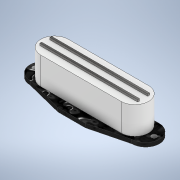
# Autodesk Inventor part: Pickup
Saved by Autodesk Inventor 2021 (Build 250183000, 183)
## iProperties
Created: 2021-02-08
Part Number: Pickup
Material: Generic
Document SubType Name: Modeling
Designer: Ryan
Density: 1 g/cm^3
Appearance: Default
Author: Ryan
Autodesk Inventor part; units mm, degrees
ref_plane "YZ Plane" through (0, 0, 0) normal (1, 0, 0) x (0, 1, 0)
ref_plane "XZ Plane" through (0, 0, 0) normal (0, 1, 0) x (-1, 0, 0)
ref_plane "XY Plane" through (0, 0, 0) normal (0, 0, 1) x (1, 0, 0)
sketch "Sketch1" plane through (0, 0, 0) normal (0, 1, 0) x (-1, 0, 0)
  line L0 (33.02, -8.89) -> (-33.02, -8.89)
  line L1 (-33.02, 8.89) -> (33.02, 8.89)
  arc A0 (33.02, -8.89) -> (33.02, 8.89) centre (33.02, 0) ccw
  arc A1 (-33.02, 8.89) -> (-33.02, -8.89) centre (-33.02, 0) ccw
  line L2 (41.91, -12.3525) -> (41.91, 10.1693) construction
  line L3 (-41.91, -12.3525) -> (-41.91, 10.1693) construction
  line L4 (8.89, 14.986) -> (-8.89, 14.986)
  line L5 (-8.89, 14.986) -> (-33.02, 8.89)
  line L6 (8.89, 14.986) -> (33.02, 8.89)
  point P0 (0, 0)
  dimension "d1" = 83.82
  dimension "d2" = 17.78
  dimension "d3" = 8.89
  dimension "d4" = 8.89
  dimension "d5" = 41.91
  dimension "d8" = 17.78
  dimension "d9" = 8.89
  dimension "d10" = 23.876
  constraints: 14 end point, 4 point on circle, 2 centre point, 2 horizontal, 2 tangent, 2 vertical, 1 equal radius, 1 parallel
  measures "d1" distance between parallel lines of L3 L2
  measures "d2" distance between parallel lines of L1 L0
  measures "d3" radius of A0
  measures "d4" distance from line of L0 point (0, 0)
  measures "d5" distance from line of L3 point (0, 0)
  measures "d8" distance of L4.start L4.end
  measures "d9" horizontal distance of point (0, 0) L4.end
  measures "d10" distance between parallel lines of L0 L4
extrude "Extrusion1" add sketch "Sketch1" along normal blind 2.54
sketch "Sketch2" plane through (0, 2.54, 0) normal (0, 1, 0) x (1, 0, 0)
  line L0 (33.02, 8.89) -> (-33.02, 8.89) projected
  line L1 (-26.035, -8.89) -> (26.035, -8.89)
  line L2 (26.035, 8.89) -> (-26.035, 8.89)
  arc A0 (-26.035, 8.89) -> (-26.035, -8.89) centre (-26.035, 0) ccw
  arc A1 (26.035, -8.89) -> (26.035, 8.89) centre (26.035, 0) ccw
  line L3 (-34.925, 8.805) -> (-34.925, -8.975) construction
  line L4 (34.925, 8.805) -> (34.925, -8.975) construction
  point P0 (0, 0)
  point P1 (-26.035, 8.89)
  dimension "d11" = 69.85
  dimension "d12" = 17.78
  dimension "d13" = 8.89
  dimension "d14" = 34.925
  constraints: 8 end point, 4 point on circle, 3 tangent, 2 centre point, 2 vertical, 1 equal radius, 1 horizontal, 1 parallel, 1 point on line
  measures "d11" distance between parallel lines of L4 L3
  measures "d12" distance between parallel lines of L0 L1
  measures "d13" radius of A0
  measures "d14" distance from line of point (0, 0) L3
extrude "Extrusion2" add sketch "Sketch2" along normal blind 17.78
sketch "Sketch3" plane through (0, 2.54, 0) normal (0, 1, 0) x (1, 0, 0)
  circle A0 centre (-38.4937, 0) radius 1.7526
  circle A1 centre (38.4937, 0) radius 1.7526
  line L0 (-40.2463, 0) -> (-41.91, 0) construction
  arc A2 (-33.02, 8.89) -> (-33.02, -8.89) centre (-33.02, 0) ccw projected
  line L1 (40.2463, 0) -> (41.91, 0) construction
  arc A3 (33.02, -8.89) -> (33.02, 8.89) centre (33.02, 0) ccw projected
  point P0 (0, 0)
  dimension "d18" = 3.5052
  dimension "d17" = 76.9874
  constraints: 4 end point, 2 horizontal alignment, 2 point on circle, 2 point on line, 1 collinear, 1 horizontal, 4 other
  measures "d17" distance of point (38.494, 0) point (-38.494, 0)
extrude "Extrusion3" cut sketch "Sketch3" against normal blind 17.78
sketch "Sketch4" plane through (0, 20.32, 0) normal (0, 1, 0) x (1, 0, 0)
  line L0 (-31.75, 3.8822) -> (31.75, 3.8822)
  line L1 (31.75, 3.8822) -> (31.75, 2.6122)
  line L2 (31.75, 2.6122) -> (-31.75, 2.6122)
  line L3 (-31.75, 2.6122) -> (-31.75, 3.8822)
  line L4 (-31.75, -2.6122) -> (31.75, -2.6122)
  line L5 (31.75, -2.6122) -> (31.75, -3.8822)
  line L6 (31.75, -3.8822) -> (-31.75, -3.8822)
  line L7 (-31.75, -3.8822) -> (-31.75, -2.6122)
  line L8 (0, 0) -> (0, 2.6122) construction
  line L9 (0, 0) -> (0, -2.6122) construction
  point P0 (0, 0)
  dimension "d21" = 63.5
  dimension "d22" = 31.75
  dimension "d23" = 1.27
  constraints: 20 end point, 4 parallel, 3 perpendicular, 3 point on line, 2 collinear, 2 horizontal, 2 midpoint, 1 coincident
  measures "d21" distance of L0.start L0.end
  measures "d22" horizontal distance of L1.end point (0, 0)
  measures "d23" distance between parallel lines of L0 L2
extrude "Extrusion4" add sketch "Sketch4" along normal blind 1.27
equation "\"d3\" = 0.5 * d2"
equation "\"d4\" = 0.5 * d2"
equation "\"d5\" = 0.5 * d1"
equation "\"d9\" = 0.5 * d8"
equation "\"d13\" = 0.5 * d12"
equation "\"d14\" = 0.5 * d11"
equation "\"d22\" = 0.5 * d21"
body "Solid1"
